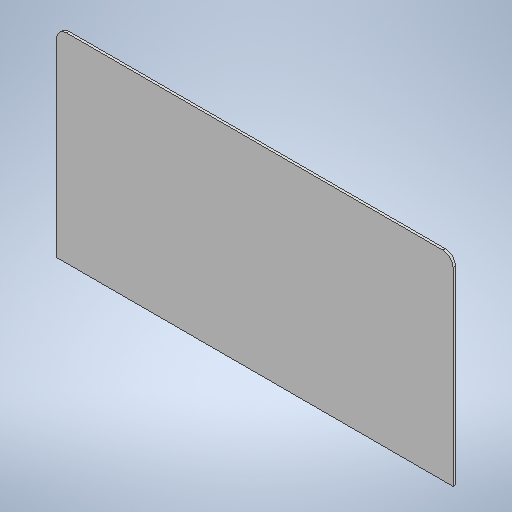
# Autodesk Inventor part: left wall
Saved by Autodesk Inventor 2025.2 (Build 292293000, 293)
## iProperties
Created: 2026-06-03
Part Number: left wall
Material: Generic
Document SubType Name: Modeling
Designer: AdminOS
Density: 1 g/cm^3
Appearance: Default
Author: AdminOS
Autodesk Inventor part; units mm, degrees
ref_plane "YZ Plane" through (0, 0, 0) normal (1, 0, 0) x (0, 1, 0)
ref_plane "XZ Plane" through (0, 0, 0) normal (0, 1, 0) x (-1, 0, 0)
ref_plane "XY Plane" through (0, 0, 0) normal (0, 0, 1) x (1, 0, 0)
sketch "Sketch1" plane through (0, 0, 0) normal (0, 0, 1) x (1, 0, 0)
  line L0 (0, 0) -> (795, 0)
  line L1 (795, 0) -> (795, 380)
  line L2 (775, 400) -> (20, 400)
  line L3 (0, 380) -> (0, 0)
  arc A0 (20, 400) -> (0, 380) centre (20, 380) ccw
  arc A1 (795, 380) -> (775, 400) centre (775, 380) ccw
  point P0 (795, 400)
  point P1 (0, 400)
  dimension "d0" = 795
  dimension "d1" = 400
  dimension "d2" = 20
  constraints: 8 end point, 4 point on circle, 4 point on line, 4 tangent, 2 centre point, 2 parallel, 1 equal radius, 1 horizontal, 1 perpendicular
  measures "d0" distance of point (0, 400) point (795, 400)
  measures "d1" distance of point (795, 400) L0.end
  measures "d2" radius of A0
extrude "Extrusion1" add sketch "Sketch1" along normal blind 5
body "Solid1"
